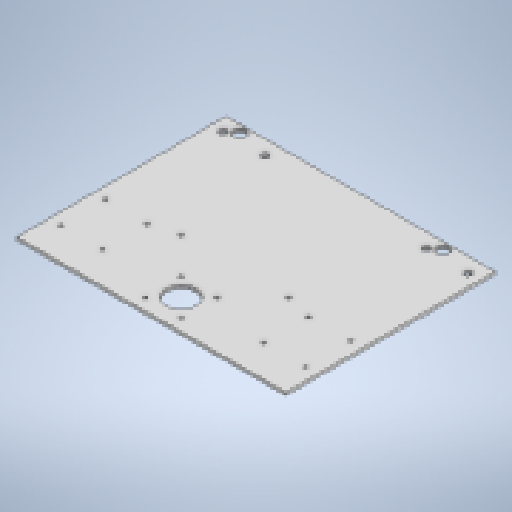
# Autodesk Inventor part: acrylic_upper
Saved by Autodesk Inventor 2026.1 (Build 301233000, 233)
## iProperties
Created: 2026-05-13
Part Number: acrylic_upper
Material: Generic
Document SubType Name: Modeling
Designer: chris
Density: 1 g/cm^3
Appearance: Default
Author: chris
Autodesk Inventor part; units mm, degrees
ref_plane "YZ Plane" through (0, 0, 0) normal (1, 0, 0) x (0, 1, 0)
ref_plane "XZ Plane" through (0, 0, 0) normal (0, 1, 0) x (-1, 0, 0)
ref_plane "XY Plane" through (0, 0, 0) normal (0, 0, 1) x (1, 0, 0)
sketch "Sketch1" plane through (0, 0, 0) normal (0, 1, 0) x (-1, 0, 0)
  line L0 (225, 175) -> (-225, 175)
  line L1 (-225, 175) -> (-225, -175)
  line L2 (-225, -175) -> (225, -175)
  line L3 (225, -175) -> (225, 175)
  line L4 (225, 175) -> (-225, -175) construction
  line L5 (-225, 175) -> (225, -175) construction
  point P0 (0, 0)
  dimension "d0" = 450
  dimension "d1" = 350
  constraints: 12 end point, 2 midpoint, 2 parallel, 1 horizontal, 1 perpendicular
  measures "d0" distance of L2.end L1.end
  measures "d1" distance of L1.end L0.end
extrude "Extrusion1" add sketch "Sketch1" along normal blind 5
sketch "Sketch2" plane through (0, 0, 0) normal (0, -1, 0) x (1, 0, 0)
  line L0 (225, 175) -> (225, -175) projected
  line L1 (-225, 175) -> (225, 175) projected
  line L2 (-225, -175) -> (-225, 175) projected
  line L3 (225, -175) -> (-225, -175) projected
  line L4 (-198.5, -164) -> (-198.5, -170) projected
  line L5 (-220, -170) -> (-198.5, -170) projected
  line L6 (-220, -115) -> (-220, -170) projected
  line L7 (-220, -115) -> (-120, -115) projected
  line L8 (-120, -115) -> (-120, -170) projected
  line L9 (-180, -170) -> (-120, -170) projected
  line L10 (-180, -170) -> (-180, -159) projected
  arc A0 (-180, -159) -> (-185, -154) centre (-185, -159) ccw projected
  line L11 (-185, -154) -> (-188.5, -154) projected
  arc A1 (-188.5, -154) -> (-198.5, -164) centre (-188.5, -164) ccw projected
  circle A2 centre (-205, -150) radius 6.1 projected
  circle A3 centre (-135, -150) radius 6.1 projected
  circle A4 centre (-205, 122) radius 3.05 projected
  circle A5 centre (-135, 47) radius 3.05 projected
  circle A6 centre (-135, 122) radius 3.05 projected
  circle A7 centre (-205, 47) radius 3.05 projected
  line L12 (-120, 134.5) -> (-120, 34.5) projected
  line L13 (-220, 34.5) -> (-120, 34.5) projected
  line L14 (-220, 134.5) -> (-220, 34.5) projected
  line L15 (-120, 134.5) -> (-220, 134.5) projected
  circle A8 centre (30, 95) radius 3.1 projected
  circle A9 centre (30, 155) radius 3.1 projected
  circle A10 centre (-30, 95) radius 3.1 projected
  circle A11 centre (-30, 155) radius 3.1 projected
  circle A12 centre (90, 215) radius 3.1 projected
  circle A13 centre (90, 35) radius 3.1 projected
  circle A14 centre (-90, 215) radius 3.1 projected
  circle A15 centre (-90, 35) radius 3.1 projected
  circle A16 centre (0, 125) radius 25 projected
  line L16 (100, 225) -> (100, 25) projected
  line L17 (100, 25) -> (-100, 25) projected
  line L18 (-100, 25) -> (-100, 225) projected
  line L19 (-100, 225) -> (100, 225) projected
  circle A17 centre (-205, -150) radius 6
  circle A18 centre (-135, -150) radius 6
  circle A19 centre (-205, 47) radius 3
  circle A20 centre (-205, 122) radius 3
  circle A21 centre (-135, 47) radius 3
  circle A22 centre (-135, 122) radius 3
  circle A23 centre (-90, 35) radius 3
  circle A24 centre (-30, 155) radius 3
  circle A25 centre (-30, 95) radius 3
  point P0 (0, 0)
  dimension "d4" = 12
  dimension "d5" = 12
  dimension "d6" = 6
  dimension "d7" = 6
  dimension "d8" = 6
  dimension "d9" = 6
  dimension "d10" = 6
  dimension "d11" = 6
  dimension "d12" = 6
  constraints: 9 centre point, 9 coincident
  measures "d4" diameter of A17
  measures "d5" diameter of A18
  measures "d6" diameter of A19
  measures "d7" diameter of A20
  measures "d8" diameter of A21
  measures "d9" diameter of A22
  measures "d10" diameter of A23
  measures "d11" diameter of A24
  measures "d12" diameter of A25
extrude "Extrusion2" cut sketch "Sketch2" against normal blind 5 contours A17 | A18 | A19 | A20 | A21 | A22 | A23 | A24 | A25
mirror "Mirror1" about plane through (0, 0, 0) normal (1, 0, 0) of "Extrusion2"
sketch "Sketch3" plane through (0, 0, 0) normal (0, -1, 0) x (1, 0, 0)
  circle A0 centre (30, 95) radius 3.1 projected
  circle A1 centre (30, 155) radius 3.1 projected
  circle A2 centre (-30, 95) radius 3.1 projected
  circle A3 centre (-30, 155) radius 3.1 projected
  circle A4 centre (90, 215) radius 3.1 projected
  circle A5 centre (90, 35) radius 3.1 projected
  circle A6 centre (-90, 215) radius 3.1 projected
  circle A7 centre (-90, 35) radius 3.1 projected
  circle A8 centre (0, 125) radius 25 projected
  line L0 (100, 225) -> (100, 25) projected
  line L1 (100, 25) -> (-100, 25) projected
  line L2 (-100, 25) -> (-100, 225) projected
  line L3 (-100, 225) -> (100, 225) projected
  point P0 (0, 0)
extrude "Extrusion3" cut sketch "Sketch3" against normal blind 5 contours A8
sketch "Sketch6" plane through (0, 5, 0) normal (0, 1, 0) x (1, 0, 0)
  circle A0 centre (0, -125) radius 25 projected
  circle A1 centre (205, -47) radius 3 projected
  circle A2 centre (90, -35) radius 3 projected
  circle A3 centre (30, -95) radius 3 projected
  circle A4 centre (205, -122) radius 3 projected
  circle A5 centre (135, 150) radius 6 projected
  circle A6 centre (135, -122) radius 3 projected
  circle A7 centre (30, -155) radius 3 projected
  circle A8 centre (135, -47) radius 3 projected
  circle A9 centre (205, 150) radius 6 projected
  circle A10 centre (-205, -47) radius 3 projected
  circle A11 centre (-90, -35) radius 3 projected
  circle A12 centre (-30, -95) radius 3 projected
  circle A13 centre (-205, -122) radius 3 projected
  circle A14 centre (-135, 150) radius 6 projected
  circle A15 centre (-135, -122) radius 3 projected
  circle A16 centre (-30, -155) radius 3 projected
  circle A17 centre (-135, -47) radius 3 projected
  circle A18 centre (-205, 150) radius 6 projected
  line L0 (225, -175) -> (225, 175) projected
  line L1 (225, 175) -> (-225, 175) projected
  line L2 (-225, 175) -> (-225, -175) projected
  line L3 (-225, -175) -> (225, -175) projected
  circle A19 centre (-189, 162) radius 10
  circle A20 centre (151, 162) radius 10
  point P0 (0, 0)
  dimension "d30" = 20
  dimension "d31" = 13
  dimension "d32" = 36
  dimension "d33" = 20
  dimension "d34" = 13
  dimension "d35" = 74
  constraints: 2 centre point
  measures "d30" diameter of A19
  measures "d31" distance from line of A19.centre L1
  measures "d32" distance from line of L2 A19.centre
  measures "d33" diameter of A20
  measures "d34" distance from line of L1 A20.centre
  measures "d35" distance from line of L0 A20.centre
extrude "Extrusion6" cut sketch "Sketch6" against normal blind 5 contours A19 | A20
body "Solid1"
